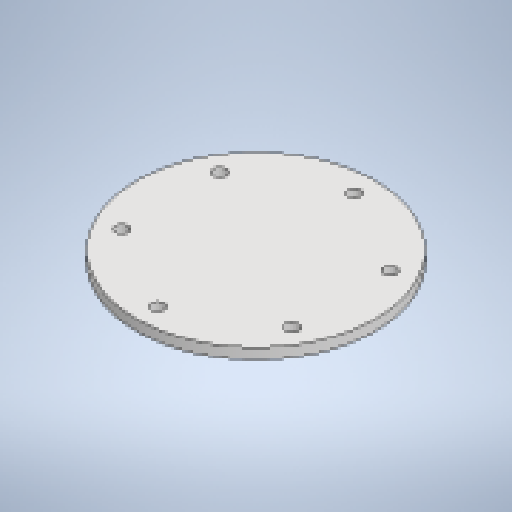
# Autodesk Inventor part: NVPH-306 revision cup
Saved by Autodesk Inventor 2025 (Build 290162010, 162A)
## iProperties
Created: 2024-04-23
Part Number: NVPH-306 revision cup
Material: Generic
Document SubType Name: Sheet Metal
Designer: user
Stock Number: ДМФ 025 кольцо прижимное корма наружное
Density: 1 g/cm^3
Sheet Metal Rule: Default
Sheet Metal Width: 225,000 mm
Sheet Metal Length: 225,000 mm
Sheet Metal Area: 50625,000 mm^2
Appearance: Default
Mass: 391.906 g
Surface Area: 875.232 cm^2
Volume: 391.906 cm^3
Flat Pattern Width: 22.5 cm
Flat Pattern Length: 22.5 cm
Flat Pattern Area: 506.25 cm^2
Author: admin
Autodesk Inventor part; units mm, degrees
ref_plane "YZ Plane" through (0, 0, 0) normal (1, 0, 0) x (0, 1, 0)
ref_plane "XZ Plane" through (0, 0, 0) normal (0, 1, 0) x (-1, 0, 0)
ref_plane "XY Plane" through (0, 0, 0) normal (0, 0, 1) x (1, 0, 0)
sketch "Sketch6" plane through (0, 0, 0) normal (0, 0, 1) x (1, 0, 0)
  circle A0 centre (0, 0) radius 72.5
  circle A1 centre (0, 0) radius 112.5
  dimension "d46" = 145
  dimension "d47" = 225
  measures "d46" diameter of A0
  measures "d47" diameter of A1
extrude "Plate1" add sketch "Sketch6" along normal blind 10 contours A0 | A1
sketch "Sketch8" plane through (0, 0, 0) normal (0, 0, -1) x (-1, 0, 0)
  circle A0 centre (0, 92.5) radius 6
  circle A1 centre (0, 0) radius 92.5 construction
  dimension "d51" = 185
  dimension "d50" = 12
  constraints: 2 vertical alignment, 1 centre point, 1 coincident, 2 other
  measures "d50" diameter of A0
extrude "Extrusion6" cut sketch "Sketch8" along normal through all both and the other way through all
pattern_circular "Circular Pattern3" count 6 over 360 about axis through (0, 0, 0) along (0, 0, 1) of "Extrusion6"
equation "\"d47\" = back_steel_circle_диам_центров + back_steel_circle_ширина_кольца"
equation "\"d51\" = back_steel_circle_диам_центров"
equation "\"d45\" = Thickness"
equation "\"BendReliefDepth\" = 0.5 * Thickness"
equation "\"back_steel_circle_диам_центров\" = 185"
equation "\"back_steel_circle_ширина_кольца\" = 40"
equation "\"Thickness\" = 10"
body "Solid2"
